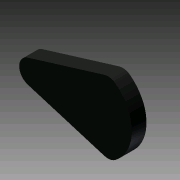
# Autodesk Inventor part: Knob 1764
Saved by Autodesk Inventor 2011 (Build 150239000, 239)
## iProperties
Created: 2010-02-22
Part Number: Knob 1764
Document SubType Name: Modeling
Designer: jgehrig
Density: 1 g/cm^3
Author: jgehrig
Autodesk Inventor part; units mm, degrees
ref_plane "YZ Plane" through (0, 0, 0) normal (1, 0, 0) x (0, 1, 0)
ref_plane "XZ Plane" through (0, 0, 0) normal (0, 1, 0) x (-1, 0, 0)
ref_plane "XY Plane" through (0, 0, 0) normal (0, 0, 1) x (1, 0, 0)
sketch "Sketch1" plane through (0, 0, 0) normal (0, 0, 1) x (1, 0, 0)
  circle A0 centre (0, 0) radius 4.445
  dimension "d0" = 8.89
  constraints: 1 centre point, 1 coincident
  measures "d0" diameter of A0
extrude "Extrusion1" add sketch "Sketch1" along normal blind 1.27
sketch "Sketch2" plane through (0, 0, 0) normal (0, 0, -1) x (-1, 0, 0)
  circle A0 centre (0, 0) radius 4.445 projected
  circle A1 centre (0, 0) radius 1.27
  dimension "d3" = 2.54
  constraints: 1 centre point, 1 coincident
  measures "d3" diameter of A1
extrude "Extrusion2" add sketch "Sketch2" along normal blind 1.27 contours A1
sketch "Sketch3" plane through (0, 0, 1.27) normal (0, 0, 1) x (1, 0, 0)
  circle A0 centre (0, 0) radius 4.445 projected
  circle A1 centre (0, 0) radius 3.175
  dimension "d6" = 6.35
  constraints: 1 centre point, 1 coincident
  measures "d6" diameter of A1
extrude "Extrusion3" add sketch "Sketch3" along normal blind 1.27 contours A1
sketch "Sketch4" plane through (0, 0, 2.54) normal (0, 0, 1) x (1, 0, 0)
  circle A0 centre (0, 0) radius 3.175 projected
  line L0 (6.35, -9.525) -> (6.35, 9.525)
  line L1 (4.9582, 9.1002) -> (-14.9068, 3.0367)
  line L2 (-14.9068, -3.0367) -> (4.9582, -9.1002)
  arc A1 (7.808, -8.5899) -> (7.808, 8.5899) centre (1.27, 0) ccw
  arc A2 (-14.9068, 3.0367) -> (-14.9068, -3.0367) centre (-13.9799, 0) ccw
  arc A3 (7.808, 8.5899) -> (4.9582, 9.1002) centre (5.8851, 6.0635) ccw
  arc A4 (4.9582, -9.1002) -> (7.808, -8.5899) centre (5.8851, -6.0635) ccw
  point P0 (-24.8555, 0)
  dimension "d9" = 19.05
  dimension "d13" = 9.525
  dimension "d14" = 6.35
  dimension "d15" = 10.795
  dimension "d16" = 3.175
  dimension "d20" = 0
  dimension "d21" = 22.225
  dimension "d22" = 3.175
  constraints: 10 point on circle, 6 end point, 6 tangent, 4 centre point, 4 point on line, 1 equal radius, 1 vertical
  measures "d9" distance of L0.start L0.end
  measures "d13" vertical distance of L0.start A0.centre
  measures "d14" distance from line of L0 A0.centre
  measures "d15" radius of A1
  measures "d16" radius of A2
  measures "d20" vertical distance of A0.centre A2.centre
  measures "d21" distance of L0.end L1.end
  measures "d22" radius of A3
extrude "Extrusion4" add sketch "Sketch4" along normal blind 3.81 contours A0 | A4 L2 A2 L1 A3 L0 | L0 A3 A1 A4
body "Solid1"
